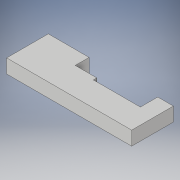
# Autodesk Inventor part: StairTemplate
Saved by Autodesk Inventor 2018.2 (Build 222227000, 227)
## iProperties
Created: 2017-12-03
Part Number: StairTemplate
Material: Generic
Document SubType Name: Modeling
Designer: steele
Density: 1 g/cm^3
Appearance: Default
Author: steele
Autodesk Inventor part; units mm, degrees
ref_plane "YZ Plane" through (0, 0, 0) normal (1, 0, 0) x (0, 1, 0)
ref_plane "XZ Plane" through (0, 0, 0) normal (0, 1, 0) x (-1, 0, 0)
ref_plane "XY Plane" through (0, 0, 0) normal (0, 0, 1) x (1, 0, 0)
sketch "Sketch1" plane through (0, 0, 0) normal (0, 1, 0) x (-1, 0, 0)
  line L0 (0, 0) -> (-228.6, 0)
  line L1 (-228.6, 0) -> (-228.6, -76.2)
  line L2 (-228.6, -76.2) -> (-200.025, -76.2)
  line L3 (-200.025, -76.2) -> (-200.025, -44.45)
  line L4 (-200.025, -44.45) -> (-114.3, -44.45)
  line L5 (-114.3, -44.45) -> (-114.3, -50.8)
  line L6 (-114.3, -50.8) -> (-74.6125, -50.8)
  line L7 (-74.6125, -50.8) -> (-74.6125, -76.2)
  line L8 (-74.6125, -76.2) -> (0, -76.2)
  line L9 (0, -76.2) -> (0, 0)
  dimension "d0" = 228.6
  dimension "d2" = 76.2
  dimension "d3" = 28.575
  dimension "d4" = 31.75
  dimension "d5" = 85.725
  dimension "d6" = 6.35
  dimension "d7" = 39.6875
  constraints: 20 end point, 5 perpendicular, 4 vertical, 1 collinear, 1 horizontal
  measures "d0" distance of L0.start L0.end
  measures "d2" distance of L0.end L1.end
  measures "d3" distance of L1.end L2.end
  measures "d4" distance of L2.end L3.end
  measures "d5" distance of L3.end L4.end
  measures "d6" distance of L4.end L5.end
  measures "d7" distance of L5.end L6.end
extrude "Extrusion1" add sketch "Sketch1" along normal blind 25.4
body "Solid1"
